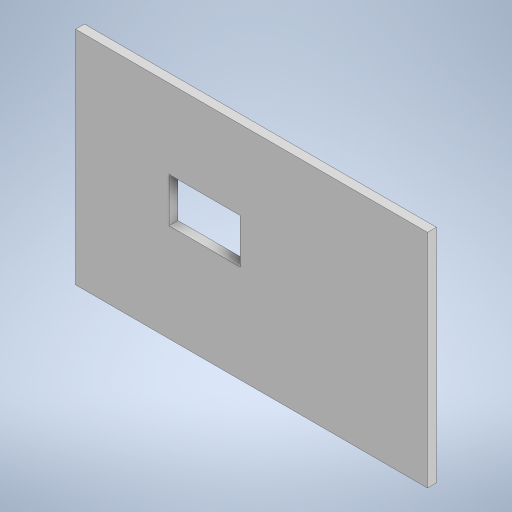
# Autodesk Inventor part: BoxCotout
Saved by Autodesk Inventor 2024.2 (Build 282272000, 272)
## iProperties
Created: 2024-08-07
Part Number: BoxCotout
Material: Generic
Document SubType Name: Modeling
Designer: UCadmin2
Density: 1 g/cm^3
Appearance: Default
Author: UCadmin2
Autodesk Inventor part; units mm, degrees
ref_plane "YZ Plane" through (0, 0, 0) normal (1, 0, 0) x (0, 1, 0)
ref_plane "XZ Plane" through (0, 0, 0) normal (0, 1, 0) x (-1, 0, 0)
ref_plane "XY Plane" through (0, 0, 0) normal (0, 0, 1) x (1, 0, 0)
sketch "Sketch1" plane through (0, 0, 0) normal (0, 0, 1) x (1, 0, 0)
  line L0 (0, 0) -> (80, 0)
  line L1 (80, 0) -> (80, 50)
  line L2 (80, 50) -> (0, 50)
  line L3 (0, 50) -> (0, 0)
  line L4 (290.5534, -110) -> (-105, -110)
  line L5 (-105, -110) -> (-105, 138.8647)
  line L6 (-105, 138.8647) -> (290.5534, 138.8647)
  line L7 (290.5534, 138.8647) -> (290.5534, -110)
  line L8 (290.5534, -110) -> (-105, 138.8647) construction
  line L9 (-105, -110) -> (290.5534, 138.8647) construction
  point P0 (92.7767, 14.4323)
  dimension "d0" = 80
  dimension "d1" = 50
  dimension "d4" = 105
  dimension "d5" = 110
  constraints: 20 end point, 4 parallel, 2 horizontal, 2 midpoint, 2 perpendicular
  measures "d0" distance of L2.end L1.end
  measures "d1" distance of L1.end L0.end
  measures "d4" distance between parallel lines of L3 L5
  measures "d5" distance between parallel lines of L0 L4
extrude "Extrusion1" add sketch "Sketch1" along normal blind 10
body "Solid1"
